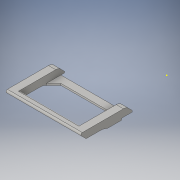
# Autodesk Inventor part: battery_clip
Saved by Autodesk Inventor 2016 (Build 200138000, 138)
## iProperties
Created: 2016-03-06
Part Number: battery_clip
Material: Generic
Document SubType Name: Modeling
Designer: dimas
Density: 1 g/cm^3
Appearance: Default
Author: dimas
Autodesk Inventor part; units mm, degrees
ref_plane "YZ Plane" through (0, 0, 0) normal (1, 0, 0) x (0, 1, 0)
ref_plane "XZ Plane" through (0, 0, 0) normal (0, 1, 0) x (-1, 0, 0)
ref_plane "XY Plane" through (0, 0, 0) normal (0, 0, 1) x (1, 0, 0)
sketch "Sketch1" plane through (0, 0, 0) normal (0, 1, 0) x (-1, 0, 0)
  line L0 (0, 0) -> (0, 76.2)
  line L1 (0, 76.2) -> (53.34, 76.2)
  line L2 (53.34, 76.2) -> (53.34, 0)
  line L3 (53.34, 0) -> (59.69, 0)
  line L4 (59.69, 0) -> (59.69, 82.55)
  line L5 (0, 0) -> (-6.35, 0)
  line L6 (-6.35, 0) -> (-6.35, 82.55)
  line L7 (-6.35, 82.55) -> (59.69, 82.55)
  dimension "d0" = 76.2
  dimension "d1" = 53.34
  dimension "d2" = 6.35
  dimension "d3" = 82.55
  dimension "d4" = 6.35
  dimension "d5" = 82.55
  constraints: 16 end point, 4 perpendicular, 3 horizontal, 1 vertical
  measures "d0" distance of L0.start L0.end
  measures "d1" distance of L0.end L1.end
  measures "d2" distance of L2.end L3.end
  measures "d3" distance of L3.end L4.end
  measures "d4" distance of L0.start L5.end
  measures "d5" distance of L5.end L6.end
extrude "Extrusion1" add sketch "Sketch1" along normal blind 6.35
sketch "Sketch2" plane through (0, 0, 0) normal (0, -1, 0) x (1, 0, 0)
  line L0 (6.35, 0) -> (0, 0) projected
  line L1 (6.35, 0) -> (6.35, 40.005)
  line L2 (6.35, 82.55) -> (6.35, 0) projected
  line L3 (-59.69, 0) -> (-59.69, 82.55) projected
  line L4 (6.35, 40.005) -> (-59.69, 40.005)
  line L5 (-59.69, 40.005) -> (-59.69, 46.355)
  line L6 (-59.69, 46.355) -> (6.35, 46.355)
  line L7 (6.35, 46.355) -> (6.35, 40.005)
  dimension "d17" = 40.005
  dimension "d18" = 6.35
  constraints: 10 end point, 2 parallel, 2 point on line, 1 horizontal, 1 perpendicular
  measures "d17" distance of L0.start L1.end
  measures "d18" distance of L4.end L5.end
extrude "Extrusion2" add sketch "Sketch2" along normal blind 1.524
sketch "Sketch3" plane through (0, -1.524, 0) normal (0, -1, 0) x (1, 0, 0)
  line L0 (-59.69, 40.005) -> (6.35, 40.005) projected
  line L1 (6.35, 40.005) -> (0, 40.005)
  line L2 (6.35, 46.355) -> (-59.69, 46.355) projected
  line L3 (0, 40.005) -> (6.35, 46.355)
  line L4 (6.35, 46.355) -> (6.35, 40.005)
  line L5 (-59.69, 40.005) -> (-59.69, 46.355)
  line L6 (-59.69, 40.005) -> (-53.34, 40.005)
  line L7 (-53.34, 40.005) -> (-59.69, 46.355)
  line L8 (6.35, 40.005) -> (6.35, 46.355)
  line L9 (6.35, 82.55) -> (6.35, 0) projected
  line L10 (6.35, 46.355) -> (0, 40.005)
  line L11 (0, 40.005) -> (6.35, 40.005)
  point P0 (0, 0)
  dimension "d21" = 6.35
  dimension "d22" = 6.35
  constraints: 18 end point, 2 collinear, 2 point on line, 1 perpendicular, 1 vertical
  measures "d21" distance of L0.end L1.end
  measures "d22" distance of L0.start L6.end
extrude "Extrusion3" cut sketch "Sketch3" against normal blind 1.524 contours L5 L7 L0 | L3 L4 L0
sketch "Sketch4" plane through (0, 0, 0) normal (0, -1, 0) x (1, 0, 0)
  line L0 (-59.69, 46.355) -> (-53.34, 40.005) projected
  line L1 (-53.34, 40.005) -> (-53.34, 36.83)
  line L2 (-53.34, 40.005) -> (-53.34, 0) projected
  line L3 (-53.34, 36.83) -> (-64.6008, 36.83)
  line L4 (-64.6008, 36.83) -> (19.5424, 36.83)
  line L5 (19.5424, 36.83) -> (19.5424, -15.2402)
  line L6 (19.5424, -15.2402) -> (-64.6008, -15.2402)
  line L7 (-64.6008, -15.2402) -> (-64.6008, 36.83)
  point P0 (0, 0)
  dimension "d25" = 3.175
  constraints: 12 end point, 2 parallel, 2 perpendicular, 1 horizontal, 1 point on line
  measures "d25" distance of L0.end L1.end
extrude "Extrusion4" cut sketch "Sketch4" against normal through all
chamfer "Chamfer4" distance 5.08 angle 45 2 edges at (-56.515, 6.35, 36.83) (3.175, 6.35, 36.83)
sketch "Sketch5" plane through (0, -1.524, 0) normal (0, -1, 0) x (1, 0, 0)
  line L0 (6.35, 46.355) -> (-59.69, 46.355) projected
  line L1 (6.35, 46.355) -> (6.35, 59.055)
  line L2 (6.35, 82.55) -> (6.35, 46.355) projected
  line L3 (6.35, 46.355) -> (-6.35, 46.355)
  line L4 (0, 46.355) -> (-53.34, 46.355) projected
  line L5 (-6.35, 46.355) -> (6.35, 59.055)
  line L6 (-59.69, 46.355) -> (-59.69, 59.055)
  line L7 (-59.69, 41.91) -> (-59.69, 82.55) projected
  line L8 (-59.69, 46.355) -> (-46.99, 46.355)
  line L9 (-46.99, 46.355) -> (-59.69, 59.055)
  point P0 (0, 0)
  dimension "d31" = 12.7
  dimension "d32" = 12.7
  dimension "d33" = 12.7
  dimension "d34" = 12.7
  constraints: 12 end point, 4 point on line
  measures "d31" distance of L0.start L1.end
  measures "d32" distance of L0.start L3.end
  measures "d33" distance of L0.end L6.end
  measures "d34" distance of L0.end L8.end
extrude "Extrusion5" add sketch "Sketch5" against normal blind 1.524
chamfer "Chamfer5" distance 5.08 angle 45 1 edges at (-26.67, 0, 82.55)
sketch "Sketch7" plane through (0, 6.35, 0) normal (0, 1, 0) x (1, 0, 0)
  point P0 (0, 0)
fillet "Fillet1" radius 6.35 2 edges at (3.175, 0, 55.88) (-56.515, 0, 55.88)
fillet "Fillet2" radius 6.35 2 edges at (-56.515, 6.35, 41.91) (3.175, 6.35, 41.91)
fillet "Fillet3" radius 1.27 2 edges at (-26.67, 6.35, 82.55) (-26.67, 5.08, 82.55)
fillet "Fillet4" radius 1.27 2 edges at (-26.67, 0, 77.47) (-26.67, 0, 76.2)
fillet "Fillet5" radius 1.27 1 edges at (-26.67, 6.35, 76.2)
body "Solid1"
